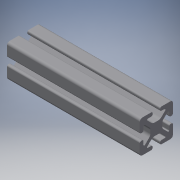
# Autodesk Inventor part: extruded aluminum
Saved by Autodesk Inventor 2017 (Build 210142000, 142)
## iProperties
Created: 2017-05-09
Part Number: extruded aluminum
Material: Generic
Document SubType Name: Modeling
Designer: slong
Density: 1 g/cm^3
Appearance: Default
Author: slong
Autodesk Inventor part; units mm, degrees
ref_plane "YZ Plane" through (0, 0, 0) normal (1, 0, 0) x (0, 1, 0)
ref_plane "XZ Plane" through (0, 0, 0) normal (0, 1, 0) x (-1, 0, 0)
ref_plane "XY Plane" through (0, 0, 0) normal (0, 0, 1) x (1, 0, 0)
sketch "Sketch1" plane through (0, 0, 0) normal (1, 0, 0) x (0, 1, 0)
  arc A0 (19.1422, -3.9768) -> (18.6646, -2.8408) centre (18.6646, -3.5092) ccw
  line L0 (15.9535, -7.2342) -> (19.1422, -3.9768)
  line L1 (21.0667, -5.7702) -> (17.9387, -8.9655)
  arc A1 (22.2128, -6.2377) -> (21.0667, -5.7702) centre (21.5444, -6.2377) ccw
  line L2 (25.0536, -2.0053) -> (25.0536, -8.7443)
  line L3 (22.2128, -8.7443) -> (22.2128, -6.2377)
  line L4 (-0.0122, -2.0053) -> (-0.0122, -8.7443)
  arc A2 (3.9747, -5.7702) -> (2.8286, -6.2377) centre (3.497, -6.2377) ccw
  arc A3 (1.9931, 0) -> (-0.0122, -2.0053) centre (1.9931, -2.0053) ccw
  line L5 (8.8992, 0) -> (1.9931, 0)
  arc A4 (7.1027, -16.4345) -> (8.0089, -14.2135) centre (4.8339, -14.2135) ccw
  arc A5 (18.6646, -22.5592) -> (19.1422, -21.4232) centre (18.6646, -21.8908) ccw
  line L6 (15.9535, -18.1658) -> (19.1422, -21.4232)
  arc A6 (21.0667, -19.6298) -> (22.2128, -19.1623) centre (21.5444, -19.1623) ccw
  line L7 (21.0667, -19.6298) -> (17.9387, -16.4345)
  line L8 (22.2128, -16.6557) -> (22.2128, -19.1623)
  line L9 (25.0536, -23.3947) -> (25.0536, -16.6557)
  line L10 (16.1422, 0) -> (23.0483, 0)
  line L11 (18.6646, -2.8408) -> (16.0299, -2.8408)
  arc A7 (22.2128, -8.7443) -> (23.3277, -9.8592) centre (23.3277, -8.7443) ccw
  line L12 (23.9387, -9.8592) -> (23.3277, -9.8592)
  arc A8 (23.9387, -9.8592) -> (25.0536, -8.7443) centre (23.9387, -8.7443) ccw
  arc A9 (6.3768, -2.8408) -> (5.8991, -3.9768) centre (6.3768, -3.5092) ccw
  line L13 (3.9747, -5.7702) -> (7.1027, -8.9655)
  line L14 (9.0879, -7.2342) -> (5.8991, -3.9768)
  arc A10 (2.8286, -19.1623) -> (3.9747, -19.6298) centre (3.497, -19.1623) ccw
  line L15 (-0.0122, -23.3947) -> (-0.0122, -16.6557)
  line L16 (3.9747, -19.6298) -> (7.1027, -16.4345)
  arc A11 (5.8991, -21.4232) -> (6.3768, -22.5592) centre (6.3768, -21.8908) ccw
  line L17 (9.0879, -18.1658) -> (5.8991, -21.4232)
  line L18 (2.8286, -16.6557) -> (2.8286, -19.1623)
  arc A12 (23.0483, -25.4) -> (25.0536, -23.3947) centre (23.0483, -23.3947) ccw
  arc A13 (25.0536, -2.0053) -> (23.0483, 0) centre (23.0483, -2.0053) ccw
  arc A14 (13.6846, -8.1882) -> (15.9535, -7.2342) centre (13.6846, -5.0132) ccw
  line L19 (13.6846, -8.1882) -> (11.3567, -8.1882)
  arc A15 (9.0115, -2.8408) -> (10.0141, -1.8382) centre (9.0115, -1.8382) ccw
  arc A16 (9.0879, -7.2342) -> (11.3567, -8.1882) centre (11.3567, -5.0132) ccw
  arc A17 (17.9387, -8.9655) -> (17.0325, -11.1865) centre (20.2075, -11.1865) ccw
  line L20 (17.0325, -14.2135) -> (17.0325, -11.1865)
  line L21 (6.3768, -2.8408) -> (9.0115, -2.8408)
  line L22 (10.0141, -1.8382) -> (10.0141, -1.1149)
  arc A18 (10.0141, -1.1149) -> (8.8992, 0) centre (8.8992, -1.1149) ccw
  line L23 (2.8286, -8.7443) -> (2.8286, -6.2377)
  arc A19 (1.7137, -9.8592) -> (2.8286, -8.7443) centre (1.7137, -8.7443) ccw
  line L24 (1.1027, -9.8592) -> (1.7137, -9.8592)
  arc A20 (-0.0122, -8.7443) -> (1.1027, -9.8592) centre (1.1027, -8.7443) ccw
  line L25 (6.3768, -22.5592) -> (9.0115, -22.5592)
  arc A21 (10.0141, -23.5618) -> (9.0115, -22.5592) centre (9.0115, -23.5618) ccw
  line L26 (10.0141, -23.5618) -> (10.0141, -24.2851)
  arc A22 (8.8992, -25.4) -> (10.0141, -24.2851) centre (8.8992, -24.2851) ccw
  line L27 (8.8992, -25.4) -> (1.9931, -25.4)
  arc A23 (17.0325, -14.2135) -> (17.9387, -16.4345) centre (20.2075, -14.2135) ccw
  line L28 (23.9387, -15.5408) -> (23.3277, -15.5408)
  arc A24 (23.3277, -15.5408) -> (22.2128, -16.6557) centre (23.3277, -16.6557) ccw
  arc A25 (25.0536, -16.6557) -> (23.9387, -15.5408) centre (23.9387, -16.6557) ccw
  line L29 (16.1422, -25.4) -> (23.0483, -25.4)
  line L30 (18.6646, -22.5592) -> (16.0299, -22.5592)
  line L31 (8.0089, -11.1865) -> (8.0089, -14.2135)
  arc A26 (8.0089, -11.1865) -> (7.1027, -8.9655) centre (4.8339, -11.1865) ccw
  arc A27 (15.0273, -1.8382) -> (16.0299, -2.8408) centre (16.0299, -1.8382) ccw
  line L32 (15.0273, -1.8382) -> (15.0273, -1.1149)
  arc A28 (16.1422, 0) -> (15.0273, -1.1149) centre (16.1422, -1.1149) ccw
  arc A29 (-0.0122, -23.3947) -> (1.9931, -25.4) centre (1.9931, -23.3947) ccw
  arc A30 (11.3567, -17.2118) -> (9.0879, -18.1658) centre (11.3567, -20.3868) ccw
  line L33 (11.3567, -17.2118) -> (13.6846, -17.2118)
  arc A31 (15.9535, -18.1658) -> (13.6846, -17.2118) centre (13.6846, -20.3868) ccw
  arc A32 (16.0299, -22.5592) -> (15.0273, -23.5618) centre (16.0299, -23.5618) ccw
  line L34 (15.0273, -23.5618) -> (15.0273, -24.2851)
  arc A33 (15.0273, -24.2851) -> (16.1422, -25.4) centre (16.1422, -24.2851) ccw
  line L35 (1.1027, -15.5408) -> (1.7137, -15.5408)
  arc A34 (1.1027, -15.5408) -> (-0.0122, -16.6557) centre (1.1027, -16.6557) ccw
  arc A35 (2.8286, -16.6557) -> (1.7137, -15.5408) centre (1.7137, -16.6557) ccw
  point P0 (0, 0)
  point P1 (12.5207, -12.7)
  dimension "d0" = 25.4
  constraints: 72 end point, 72 point on circle, 36 centre point
  measures "d0" distance between parallel lines of L29 L10
extrude "Extrusion1" add sketch "Sketch1" along normal blind 101.6
body "Solid1"
